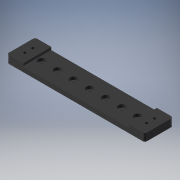
# Autodesk Inventor part: Sensor Calibration Rail Wall Support
Saved by Autodesk Inventor 2019 (Build 230136000, 136)
## iProperties
Created: 2019-01-19
Part Number: Sensor Calibration Rail Wall Support
Material: Generic
Document SubType Name: Modeling
Designer: Billy
Density: 1 g/cm^3
Appearance: Default
Author: Billy
Autodesk Inventor part; units mm, degrees
ref_plane "YZ Plane" through (0, 0, 0) normal (1, 0, 0) x (0, 1, 0)
ref_plane "XZ Plane" through (0, 0, 0) normal (0, 1, 0) x (-1, 0, 0)
ref_plane "XY Plane" through (0, 0, 0) normal (0, 0, 1) x (1, 0, 0)
sketch "Sketch1" plane through (0, 0, 0) normal (0, 1, 0) x (-1, 0, 0)
  circle A0 centre (51, 2.5) radius 2
  circle A1 centre (51, 12.5) radius 2
  circle A2 centre (-101, 12.5) radius 2
  circle A3 centre (-101, 2.5) radius 2
  line L0 (-106, -5) -> (56, -5)
  line L1 (56, -5) -> (56, 20)
  line L2 (-106, 20) -> (56, 20)
  line L3 (-50, 20) -> (-106, 20)
  line L4 (-106, 20) -> (-106, -5)
  point P0 (0, 0)
  point P1 (0, -5)
  constraints: 10 end point, 4 centre point
extrude "Extrusion1" add sketch "Sketch1" along normal blind 5
sketch "Sketch2" plane through (0, 5, 0) normal (0, 1, 0) x (1, 0, 0)
  circle A0 centre (101, -2.5) radius 2 projected
  circle A1 centre (101, -12.5) radius 2 projected
  circle A2 centre (-51, -12.5) radius 2 projected
  circle A3 centre (-51, -2.5) radius 2 projected
  line L0 (106, 5) -> (-56, 5) projected
  line L1 (-56, 5) -> (-56, -20) projected
  line L2 (-56, -20) -> (106, -20) projected
  line L3 (106, -20) -> (106, 5) projected
  line L4 (106, 5) -> (-56, 5) projected
  line L5 (-56, -20) -> (-46, -20)
  line L6 (-46, -20) -> (-46, 5)
  line L7 (-46, 5) -> (-56, 5)
  line L8 (-56, 5) -> (-56, -20)
  line L9 (106, -20) -> (106, 5) projected
  line L10 (106, -20) -> (96, -20)
  line L11 (96, -20) -> (96, 5)
  line L12 (96, 5) -> (106, 5)
  line L13 (106, 5) -> (106, -20)
  point P0 (0, 0)
  dimension "d2" = 10
  dimension "d3" = 10
  constraints: 16 end point, 4 parallel, 2 horizontal, 2 perpendicular, 2 point on line
  measures "d2" distance of L7.end L6.end
  measures "d3" distance of L11.end L12.end
extrude "Extrusion2" add sketch "Sketch2" along normal blind 3.5 contours L3 L2 L11 L0 | L6 L2 L1 L0
sketch "Sketch3" plane through (0, 5, 0) normal (0, 1, 0) x (1, 0, 0)
  line L0 (-46, 5) -> (-46, -20) projected
  line L1 (-46, -20) -> (96, -20) projected
  line L2 (96, -20) -> (96, 5) projected
  line L3 (96, 5) -> (-46, 5) projected
  circle A0 centre (25, -7.5) radius 2
  circle A1 centre (45, -7.5) radius 2
  circle A2 centre (65, -7.5) radius 2
  circle A3 centre (85, -7.5) radius 2
  circle A4 centre (5, -7.5) radius 2
  circle A5 centre (25, -7.5) radius 2
  circle A6 centre (45, -7.5) radius 2
  circle A7 centre (65, -7.5) radius 2
  circle A8 centre (-15, -7.5) radius 2
  circle A9 centre (5, -7.5) radius 2
  circle A10 centre (25, -7.5) radius 2
  circle A11 centre (45, -7.5) radius 2
  circle A12 centre (-35, -7.5) radius 2
  circle A13 centre (-15, -7.5) radius 2
  circle A14 centre (5, -7.5) radius 2
  circle A15 centre (25, -7.5) radius 2
  point P0 (0, 0)
  dimension "d6" = 4
  dimension "d9" = 20
  dimension "d12" = 20
  constraints: 16 centre point, 2 horizontal, 30 other
  measures "d6" diameter of A0
  measures "d9" distance of A0.centre A1.centre
  measures "d12" distance of A0.centre A4.centre
extrude "Extrusion3" cut sketch "Sketch3" against normal blind 5 contours A0 | A1 | A2 | A3 | A4 | A8 | A12
sketch "Sketch4" plane through (0, 5, 0) normal (0, 1, 0) x (1, 0, 0)
  circle A0 centre (-15, -7.5) radius 2 projected
  circle A1 centre (85, -7.5) radius 2 projected
  circle A2 centre (45, -7.5) radius 2 projected
  circle A3 centre (25, -7.5) radius 2 projected
  circle A4 centre (65, -7.5) radius 2 projected
  circle A5 centre (5, -7.5) radius 2 projected
  circle A6 centre (-35, -7.5) radius 2 projected
  line L0 (-46, 5) -> (-46, -20) projected
  line L1 (-46, -20) -> (96, -20) projected
  line L2 (96, -20) -> (96, 5) projected
  line L3 (96, 5) -> (-46, 5) projected
  circle A7 centre (-35, -7.5) radius 5
  circle A8 centre (-15, -7.5) radius 5
  circle A9 centre (5, -7.5) radius 5
  circle A10 centre (25, -7.5) radius 5
  circle A11 centre (45, -7.5) radius 5
  circle A12 centre (65, -7.5) radius 5
  circle A13 centre (85, -7.5) radius 5
  point P0 (0, 0)
  dimension "d17" = 10
  dimension "d18" = 10
  dimension "d19" = 10
  dimension "d20" = 10
  dimension "d21" = 10
  dimension "d22" = 10
  dimension "d23" = 10
  constraints: 7 centre point, 1 coincident
  measures "d17" diameter of A7
  measures "d18" diameter of A8
  measures "d19" diameter of A9
  measures "d20" diameter of A10
  measures "d21" diameter of A11
  measures "d22" diameter of A12
  measures "d23" diameter of A13
extrude "Extrusion4" cut sketch "Sketch4" against normal blind 4 contours A7 | A8 | A9 | A10 | A11 | A12 | A13
move faces "Move1" translate (0, -1, 0) faces at (25.0804, 0, -1.4951)
move faces "Move2" translate (-5, 0, 0) faces at (-56, 5.3333, 3.3333)
move faces "Move3" translate (5, 0, 0) faces at (106, 2.1667, 3.3333)
move faces "Move4" translate (0, 0, 5) faces at (1.3333, 1, 20)
move faces "Move5" translate (0, 0, -5) faces at (48.6667, 1, -5)
fillet "Fillet1" radius 2.5 4 edges at (111, 3.75, -10) (111, 3.75, 25) (-61, 3.75, -10) (-61, 3.75, 25)
move faces "Move6" translate (-5, 0, 0) faces at (96, 6.1667, 13.3333)
move faces "Move7" translate (5, 0, 0) faces at (-46, 6.1667, 13.3333)
sketch "Sketch5" plane through (-58.5, -1, -10) normal (0, -1, 0) x (1, 0, 0)
  arc A0 (0, 35) -> (-2.5, 32.5) centre (0, 32.5) ccw projected
  line L0 (-2.5, 2.5) -> (-2.5, 32.5) projected
  arc A1 (-2.5, 2.5) -> (0, 0) centre (0, 2.5) ccw projected
  line L1 (167, 0) -> (0, 0) projected
  arc A2 (167, 0) -> (169.5, 2.5) centre (167, 2.5) ccw projected
  line L2 (169.5, 32.5) -> (169.5, 2.5) projected
  arc A3 (169.5, 32.5) -> (167, 35) centre (167, 32.5) ccw projected
  line L3 (0, 35) -> (167, 35) projected
  circle A4 centre (43.5, 17.5) radius 2 projected
  circle A5 centre (143.5, 17.5) radius 2 projected
  circle A6 centre (103.5, 17.5) radius 2 projected
  circle A7 centre (83.5, 17.5) radius 2 projected
  circle A8 centre (123.5, 17.5) radius 2 projected
  circle A9 centre (63.5, 17.5) radius 2 projected
  circle A10 centre (23.5, 17.5) radius 2 projected
  circle A11 centre (159.5, 12.5) radius 2 projected
  circle A12 centre (159.5, 22.5) radius 2 projected
  circle A13 centre (7.5, 22.5) radius 2 projected
  circle A14 centre (7.5, 12.5) radius 2 projected
  arc A15 (154.5, 12.5) -> (164.5, 12.5) centre (159.5, 12.5) ccw
  arc A16 (164.5, 22.5) -> (154.5, 22.5) centre (159.5, 22.5) ccw
  arc A17 (2.5, 12.5) -> (12.5, 12.5) centre (7.5, 12.5) ccw
  arc A18 (12.5, 22.5) -> (2.5, 22.5) centre (7.5, 22.5) ccw
  line L4 (164.5, 12.5) -> (164.5, 22.5)
  line L5 (154.5, 12.5) -> (154.5, 22.5)
  line L6 (12.5, 12.5) -> (12.5, 22.5)
  line L7 (2.5, 12.5) -> (2.5, 22.5)
  point P0 (58.5, 10)
  dimension "d48" = 10
  dimension "d49" = 10
  dimension "d50" = 10
  dimension "d51" = 10
  constraints: 8 end point, 8 point on circle, 4 centre point, 3 tangent, 1 coincident, 1 vertical
  measures "d48" diameter of A15
  measures "d49" diameter of A16
  measures "d50" diameter of A17
  measures "d51" diameter of A18
extrude "Extrusion5" cut sketch "Sketch5" against normal blind 4 contours L5 A16 L4 A15 | L7 A18 L6 A17
body "Solid1"
